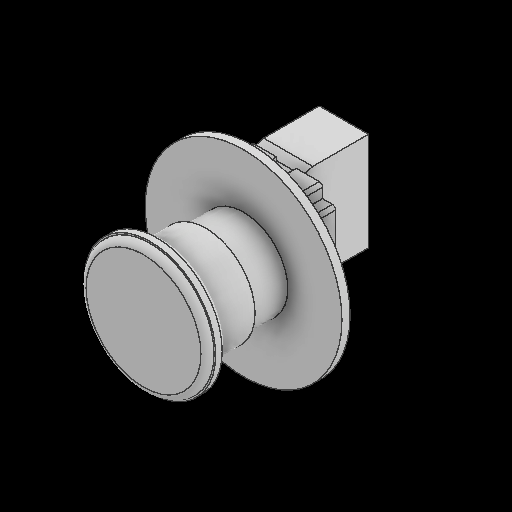
# Autodesk Inventor part: E-Stop
Saved by Autodesk Inventor 2025.2 (Build 292293000, 293)
## iProperties
Created: 2026-05-14
Part Number: E-Stop
Material: Generic
Document SubType Name: Modeling
Designer: valer
Density: 1 g/cm^3
Appearance: Default
Author: valer
Autodesk Inventor part; units mm, degrees
ref_plane "YZ Plane" through (0, 0, 0) normal (1, 0, 0) x (0, 1, 0)
ref_plane "XZ Plane" through (0, 0, 0) normal (0, 1, 0) x (-1, 0, 0)
ref_plane "XY Plane" through (0, 0, 0) normal (0, 0, 1) x (1, 0, 0)
sketch "Base" plane through (0, 0, 0) normal (0, 0, 1) x (1, 0, 0)
  line L0 (-15, -20) -> (15, -20)
  line L1 (15, -20) -> (15, 20)
  line L2 (15, 20) -> (-15, 20)
  line L3 (-15, 20) -> (-15, -20)
  line L4 (-15, -20) -> (15, 20) construction
  line L5 (15, -20) -> (-15, 20) construction
  circle A0 centre (0, 0) radius 11.125
  line L6 (-15, 20) -> (-11, 20)
  line L7 (-11, 20) -> (-11, 16)
  line L8 (-11, 16) -> (-15, 16)
  line L9 (-15, 16) -> (-15, 20)
  line L10 (-21, 0) -> (21, 0) construction
  line L11 (0, -28) -> (0, 28) construction
  line L12 (11, 20) -> (11, 16)
  line L13 (11, 16) -> (15, 16)
  line L14 (-11, -20) -> (-11, -16)
  line L15 (-11, -16) -> (-15, -16)
  line L16 (11, -16) -> (15, -16)
  line L17 (11, -20) -> (11, -16)
  dimension "d0" = 40
  dimension "d1" = 30
  dimension "d2" = 22.25
  dimension "d5" = 4
  constraints: 32 end point, 9 symmetric about line, 4 parallel, 3 perpendicular, 2 horizontal, 2 midpoint, 1 centre point, 1 coincident
  measures "d0" distance of L2.end L0.start
  measures "d1" distance of L1.end L2.end
  measures "d2" diameter of A0
  measures "d5" distance of L6.end L7.end
extrude "BaseFeature" add sketch "Base" along normal blind 10.6 contours L14 L15 L3 L8 L7 L2 L12 L13 L1 L16 L17 L0
fillet "BaseFilletsFeature" radius 1 11 edges at (-15, 16, 5.3) (-11, 20, 5.3) (11, 20, 5.3) (15, 16, 5.3) (-11, 16, 5.3) (-15, -16, 5.3) (-11, -16, 5.3) (-11, -20, 5.3) (11, -20, 5.3) (11, -16, 5.3) (15, -16, 5.3)
sketch "MountHoles" plane through (0, 0, 10.6) normal (0, 0, 1) x (1, 0, 0)
  line L0 (10, 20) -> (-10, 20) projected
  line L1 (-3, 20) -> (3, 20)
  line L2 (3, 20) -> (3, 19)
  line L3 (3, 19) -> (-3, 19)
  line L4 (-3, 19) -> (-3, 20)
  line L5 (-21, 0) -> (21, 0) construction
  line L6 (3, -20) -> (3, -19)
  line L7 (3, -19) -> (-3, -19)
  line L8 (-3, -19) -> (-3, -20)
  line L9 (-10, -20) -> (10, -20) projected
  circle A0 centre (0, 0) radius 11.125 construction
  circle A1 centre (0, 15) radius 2
  circle A2 centre (0, -15) radius 2
  line L10 (0, -28) -> (0, 28) construction
  point P0 (0, 20)
  dimension "d7" = 1
  dimension "d8" = 6
  dimension "d9" = 4
  dimension "d10" = 30
  constraints: 14 end point, 5 symmetric about line, 2 centre point, 2 midpoint, 2 parallel, 2 point on line, 1 horizontal, 1 perpendicular, 1 other
  measures "d7" distance of L1.end L2.end
  measures "d8" distance of L2.end L3.end
  measures "d9" diameter of A1
  measures "d10" distance of A2.centre A1.centre
extrude "MountHolesFeature" cut sketch "MountHoles" against normal through all
sketch "Body" plane through (0, 0, 0) normal (0, 0, -1) x (-1, 0, 0)
  line L0 (15, 15) -> (0, 15)
  line L1 (0, 15) -> (0, -15)
  line L2 (0, -15) -> (15, -15)
  line L3 (15, -15) -> (15, 15)
  line L4 (15, 15) -> (15, -15) projected
  point P0 (0, 0)
  dimension "d13" = 15
  constraints: 8 end point, 2 parallel, 1 collinear, 1 horizontal, 1 perpendicular
  measures "d13" distance of L0.start L0.end
extrude "BodyFeature" add sketch "Body" along normal blind 25
sketch "Chamfer" plane through (-15, -15, 10.6) normal (-1, 0, 0) x (0, 0, 1)
  line L0 (-10.6, 0) -> (-35.6, 0) projected
  line L1 (-10.6, 0) -> (-10.6, 2.3)
  line L2 (-10.6, 0) -> (-10.6, 30) projected
  line L3 (-10.6, 2.3) -> (-18.6, 0)
  line L4 (-42.72, 15) -> (7.12, 15) construction
  line L5 (-10.6, 30) -> (-10.6, 27.7)
  line L6 (-10.6, 27.7) -> (-18.6, 30)
  line L7 (-10.6, 30) -> (-35.6, 30) projected
  line L8 (-18.6, 30) -> (-18.6, 0) construction
  point P0 (-10.6, 15)
  dimension "d16" = 8
  dimension "d17" = 2.3
  constraints: 10 end point, 2 point on line, 2 symmetric about line, 1 perpendicular
  measures "d16" distance between parallel lines of L2 L8
  measures "d17" distance of L0.start L1.end
extrude "ChamferFeature" cut sketch "Chamfer" against normal through all
sketch "Terminals" plane through (0, 0, -25) normal (0, 0, -1) x (-1, 0, 0)
  line L0 (15, -15) -> (15, 15) construction
  line L1 (15, 15) -> (0, 15) construction
  line L2 (0, 15) -> (0, -15) construction
  line L3 (0, -15) -> (15, -15) construction
  line L4 (0, -15) -> (15, -15) projected
  line L5 (5.7, -15) -> (5.7, 15) construction
  line L6 (21, 0) -> (-21, 0) construction
  line L7 (5.7, -12.59) -> (8.87, -12.59)
  line L8 (8.87, -12.59) -> (8.87, -6.25) construction
  line L9 (8.87, -6.25) -> (5.7, -6.25)
  line L10 (5.7, -6.25) -> (5.7, -12.59)
  circle A0 centre (8.87, -9.42) radius 3.17
  line L11 (8.87, -9.42) -> (12.04, -9.42) construction
  line L12 (5.7, 12.59) -> (8.87, 12.59)
  line L13 (8.87, 6.25) -> (5.7, 6.25)
  line L14 (5.7, 6.25) -> (5.7, 12.59)
  circle A1 centre (8.87, 9.42) radius 3.17
  line L15 (5.7, -3.5) -> (9.4, -3.5)
  line L16 (9.4, -3.5) -> (9.4, 3.5)
  line L17 (9.4, 3.5) -> (5.7, 3.5)
  line L18 (5.7, 3.5) -> (5.7, -3.5)
  point P0 (0, 0)
  point P1 (5.7, 0)
  dimension "d20" = 6.34
  dimension "d21" = 5.7
  dimension "d22" = 12.5
  dimension "d23" = 3.7
  dimension "d24" = 7
  constraints: 26 end point, 5 point on line, 5 symmetric about line, 4 parallel, 3 horizontal, 3 perpendicular, 2 midpoint, 2 point on circle, 1 centre point, 1 tangent, 4 other
  measures "d20" distance between parallel lines of L9 L7
  measures "d21" distance between parallel lines of L2 L5
  measures "d22" distance between parallel lines of L13 L9
  measures "d23" distance of L15.start L15.end
  measures "d24" distance of L15.end L16.end
extrude "TerminalsFeature" cut sketch "Terminals" against normal blind 10
sketch "Ring" plane through (0, 0, 10.6) normal (0, 0, 1) x (1, 0, 0)
  arc A0 (0, -11.125) -> (0, 11.125) centre (0, 0) ccw projected
  circle A1 centre (0, 0) radius 30
  circle A2 centre (0, 0) radius 11.25
  dimension "d27" = 60
  dimension "d28" = 22.5
  constraints: 2 centre point, 2 coincident
  measures "d27" diameter of A1
  measures "d28" diameter of A2
extrude "RingFeature" add sketch "Ring" along normal blind 2.5
sketch "ButtonNeck" plane through (0, 0, 13.1) normal (0, 0, 1) x (1, 0, 0)
  arc A0 (0, -11.125) -> (0, 11.125) centre (0, 0) ccw projected
  circle A1 centre (0, 0) radius 13.5
  dimension "d31" = 27
  constraints: 1 centre point, 1 coincident
  measures "d31" diameter of A1
extrude "ButtonNeckFeature" add sketch "ButtonNeck" along normal blind 11.5
sketch "ButtonBody" plane through (0, 0, 24.6) normal (0, 0, 1) x (1, 0, 0)
  circle A0 centre (0, 0) radius 11.25 projected
  circle A1 centre (0, 0) radius 15
  dimension "d34" = 30
  constraints: 1 centre point, 1 coincident
  measures "d34" diameter of A1
extrude "ButtonBodyFeature" add sketch "ButtonBody" along normal blind 13 contours A0 | A1
sketch "ButtonHead" plane through (0, 0, 0) normal (0, 1, 0) x (-1, 0, 0)
  line L0 (15, 37.6) -> (-15, 37.6) projected
  line L1 (-15, 37.6) -> (-19.5, 37.6)
  line L2 (-19.5, 37.6) -> (-19.5, 39.6)
  line L3 (-19.5, 39.6) -> (-20, 39.6)
  line L4 (-20, 39.6) -> (-20, 41.6)
  line L5 (-20, 41.6) -> (-19.5, 41.6)
  line L6 (-19.5, 41.6) -> (-19.5, 43.6)
  line L7 (-19.5, 43.6) -> (0, 43.6)
  line L8 (0, 43.6) -> (0, 37.6)
  line L9 (-20, 40.6) -> (0, 40.6) construction
  line L10 (0, -38.72) -> (0, 57.32) projected
  point P0 (0, 0)
  point P1 (-17.25, 37.6)
  dimension "d37" = 6
  dimension "d38" = 2
  dimension "d39" = 20
  dimension "d40" = 0.5
  constraints: 18 end point, 6 perpendicular, 4 midpoint, 2 point on line, 1 horizontal
  measures "d37" distance from line of point (-17.25, 37.6) L7
  measures "d38" distance of L3.end L4.end
  measures "d39" distance between parallel lines of L8 L4
  measures "d40" distance of L2.end L3.end
revolve "ButtonHeadFeature" add sketch "ButtonHead" angle 360 about axis through (0, 0, -10) along (0, 0, 1)
fillet "ButtonHeadFilletsFeature" radius 2 3 edges at (-15, 0, 37.6) (-19.5, 0, 37.6) (-19.5, 0, 43.6)
body "Solid1"
